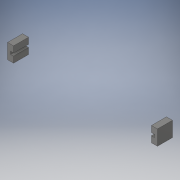
# Autodesk Inventor part: CardRailStandard
Saved by Autodesk Inventor 2018 (Build 220112000, 112)
## iProperties
Created: 2018-01-15
Part Number: CardRailStandard
Material: Aluminum
Document SubType Name: Modeling
Designer: Bradley
Density: 2.7 g/cm^3
Appearance: Anodized - Light Gray
Author: Bradley
Revision Number: 3.1
Autodesk Inventor part; units mm, degrees
ref_plane "YZ Plane" through (0, 0, 0) normal (1, 0, 0) x (0, 1, 0)
ref_plane "XZ Plane" through (0, 0, 0) normal (0, 1, 0) x (-1, 0, 0)
ref_plane "XY Plane" through (0, 0, 0) normal (0, 0, 1) x (1, 0, 0)
sketch "Sketch1" plane through (0, 0, 0) normal (0, 0, 1) x (1, 0, 0)
  line L0 (-46, 5) -> (-46, 0.9)
  line L1 (-46, 0.9) -> (-48, 0.9)
  line L2 (-48, 0.9) -> (-48, -0.9)
  line L3 (-48, -0.9) -> (-46, -0.9)
  line L4 (-46, -0.9) -> (-46, -5)
  line L5 (-46, -5) -> (-50, -5)
  line L6 (-50, -5) -> (-50, 5)
  line L7 (-50, 5) -> (-46, 5)
  line L8 (0, 5) -> (0, -5)
  line L9 (46, 5) -> (46, 0.9)
  line L10 (46, 0.9) -> (48, 0.9)
  line L11 (48, 0.9) -> (48, -0.9)
  line L12 (48, -0.9) -> (46, -0.9)
  line L13 (46, -0.9) -> (46, -5)
  line L14 (46, -5) -> (50, -5)
  line L15 (50, -5) -> (50, 5)
  line L16 (50, 5) -> (46, 5)
  point P0 (0, 0)
  point P1 (-48, 0)
  point P2 (-50, 0)
  dimension "d0" = 100
  dimension "d1" = 2
  dimension "d2" = 96
  dimension "d3" = 4
  dimension "d4" = 1.8
  dimension "d5" = 10
  dimension "d6" = 2
  dimension "d7" = 92
  constraints: 34 end point, 8 symmetric about line, 7 perpendicular, 6 point on line, 3 midpoint, 2 horizontal alignment, 1 vertical
  measures "d0" distance between parallel lines of L15 L6
  measures "d1" distance between parallel lines of L6 L2
  measures "d2" distance between parallel lines of L11 L2
  measures "d3" distance between parallel lines of L6 L4
  measures "d4" distance of L1.end L2.end
  measures "d5" distance of L5.end L6.end
  measures "d6" distance of L0.end L1.end
  measures "d7" distance between parallel lines of L9 L0
extrude "Extrusion1" add sketch "Sketch1" along normal mid plane 10
body "Solid1"
